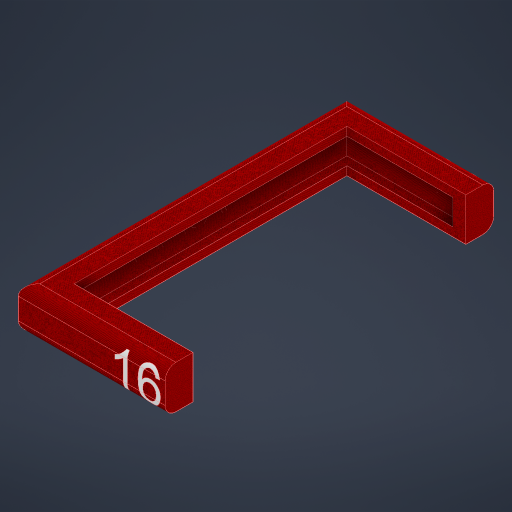
# Autodesk Inventor part: BUMP_005_BumperCloth
Saved by Autodesk Inventor 2024.2 (Build 282272000, 272)
## iProperties
Created: 2024-08-07
Part Number: BUMP_005_BumperCloth
Material: 1000 Denier Nylon Cordura
Document SubType Name: Modeling
Designer: Bryan
Density: 1 g/cm^3
Appearance: Default(1)
Mass: 229.5 g
Surface Area: 11381.8 cm^2
Volume: 229.5 cm^3
Author: Bryan
Autodesk Inventor part; units mm, degrees
ref_plane "YZ Plane" through (0, 0, 0) normal (1, 0, 0) x (0, 1, 0)
ref_plane "XZ Plane" through (0, 0, 0) normal (0, 1, 0) x (-1, 0, 0)
ref_plane "XY Plane" through (0, 0, 0) normal (0, 0, 1) x (1, 0, 0)
sketch "Sketch2" plane through (0, 0, 0) normal (1, 0, 0) x (0, 1, 0)
  line L0 (127, 0) -> (127, -82.55) construction
  line L1 (127, -82.55) -> (0, -82.55) construction
  line L2 (0, -82.55) -> (0, 0) construction
  circle A0 centre (95.25, -50.8) radius 31.75 construction
  circle A1 centre (31.75, -50.8) radius 31.75 construction
  arc A2 (95.25, -82.55) -> (127, -50.8) centre (95.25, -50.8) ccw
  arc A3 (0, -50.8) -> (31.75, -82.55) centre (31.75, -50.8) ccw
  line L3 (31.75, -82.55) -> (95.25, -82.55)
  line L4 (0, -50.8) -> (0, 0)
  line L5 (127, -50.8) -> (127, 0)
  line L6 (127, 0) -> (101.6, 0)
  line L7 (0, 0) -> (25.4, 0)
  line L8 (101.6, 0.4) -> (127.4, 0.4)
  line L9 (127.4, 0.4) -> (127.4, -50.8)
  arc A4 (95.25, -82.95) -> (127.4, -50.8) centre (95.25, -50.8) ccw
  line L10 (95.25, -82.95) -> (31.75, -82.95)
  arc A5 (-0.4, -50.8) -> (31.75, -82.95) centre (31.75, -50.8) ccw
  line L11 (-0.4, -50.8) -> (-0.4, 0.4)
  line L12 (-0.4, 0.4) -> (25.4, 0.4)
  line L13 (127, 0) -> (0, -82.55) construction
  line L14 (0, 0) -> (127, -82.55) construction
  line L15 (101.6, 0.4) -> (101.6, 0)
  line L16 (25.4, 0.4) -> (25.4, 0)
  point P0 (63.5, -41.275)
  dimension "d1" = 82.55
  dimension "d2" = 127
  dimension "d3" = 63.5
  dimension "d4" = 25.4
  dimension "d5" = 25.4
  dimension "d6" = 127
  dimension "d7" = 0.4
  constraints: 34 end point, 12 point on circle, 7 tangent, 6 centre point, 4 point on line, 4 vertical, 3 concentric, 3 horizontal, 1 equal radius, 1 midpoint, 1 parallel, 6 other
  measures "d1" distance of L0.start L0.end
  measures "d2" distance of L2.end L0.start
  measures "d3" diameter of A0
  measures "d4" distance of L0.start L6.end
  measures "d5" distance of L2.end L7.end
  measures "d6" distance of L0.end L1.end
  measures "d7" distance between parallel lines of L6 L8
sketch3d "3D Sketch1"
  line L0 (0, 63.5, -41.275) -> (-395.2875, 63.5, -41.275)
  line L1 (-395.2875, 63.5, -41.275) -> (-395.2875, 63.5, 854.075)
  line L2 (-395.2875, 63.5, 854.075) -> (0, 63.5, 854.075)
  dimension "d10" = 395.2875
  dimension "d11" = 895.35
sweep "Sweep1" add profiles "Sketch2" path "3D Sketch1"
sketch "Sketch3" plane through (0, 31.75, 895.35) normal (1, 0, 0) x (0, 0, -1)
  line L0 (895.35, -31.75) -> (895.35, -6.35) projected
  line L1 (895.35, -6.35) -> (894.95, -6.35) projected
  line L2 (894.95, -6.35) -> (894.95, -32.15) projected
  line L3 (894.95, -32.15) -> (946.15, -32.15) projected
  arc A0 (946.15, -32.15) -> (978.3, 0) centre (946.15, 0) ccw projected
  line L4 (978.3, 0) -> (978.3, 63.5) projected
  arc A1 (978.3, 63.5) -> (946.15, 95.65) centre (946.15, 63.5) ccw projected
  line L5 (946.15, 95.65) -> (894.95, 95.65) projected
  line L6 (894.95, 95.65) -> (894.95, 69.85) projected
  line L7 (894.95, 69.85) -> (895.35, 69.85) projected
  line L8 (895.35, 69.85) -> (895.35, 95.25) projected
  line L9 (895.35, 95.25) -> (946.15, 95.25) projected
  arc A2 (977.9, 63.5) -> (946.15, 95.25) centre (946.15, 63.5) ccw projected
  line L10 (977.9, 63.5) -> (977.9, 0) projected
  arc A3 (946.15, -31.75) -> (977.9, 0) centre (946.15, 0) ccw projected
  line L11 (946.15, -31.75) -> (895.35, -31.75) projected
  line L12 (894.95, 69.85) -> (894.95, -6.35)
  line L13 (82.55, -6.35) -> (82.55, -31.75) projected
  line L14 (82.55, -31.75) -> (31.75, -31.75) projected
  arc A4 (0, 0) -> (31.75, -31.75) centre (31.75, 0) ccw projected
  line L15 (0, 0) -> (0, 63.5) projected
  arc A5 (31.75, 95.25) -> (0, 63.5) centre (31.75, 63.5) ccw projected
  line L16 (31.75, 95.25) -> (82.55, 95.25) projected
  line L17 (82.55, 95.25) -> (82.55, 69.85) projected
  line L18 (82.55, 69.85) -> (82.95, 69.85) projected
  line L19 (82.95, 69.85) -> (82.95, 95.65) projected
  line L20 (82.95, 95.65) -> (31.75, 95.65) projected
  arc A6 (31.75, 95.65) -> (-0.4, 63.5) centre (31.75, 63.5) ccw projected
  line L21 (-0.4, 63.5) -> (-0.4, 0) projected
  arc A7 (-0.4, 0) -> (31.75, -32.15) centre (31.75, 0) ccw projected
  line L22 (31.75, -32.15) -> (82.95, -32.15) projected
  line L23 (82.95, -32.15) -> (82.95, -6.35) projected
  line L24 (82.95, -6.35) -> (82.55, -6.35) projected
  line L25 (82.95, 69.85) -> (82.95, -6.35)
  constraints: 4 end point, 2 vertical
extrude "Extrusion1" add sketch "Sketch3" along normal blind 0.4
sketch "Sketch4" plane through (-353.6125, 101.6, 812.4) normal (0, 0, -1) x (-1, 0, 0)
  line L0 (0, 0) -> (-353.6125, 0) projected
  line L1 (-353.6125, -76.2) -> (-353.6125, 0) projected
  line L2 (0, -76.2) -> (-353.6125, -76.2) projected
  line L3 (-315.5125, 0) -> (-315.5125, -76.2)
  point P0 (-353.6125, -101.6)
  dimension "d16" = 38.1
  constraints: 2 end point, 2 point on line, 1 vertical
  measures "d16" distance between parallel lines of L1 L3
extrude "Extrusion2" add sketch "Sketch4" against normal blind 0.4
sketch "Sketch6" plane through (0, 31.75, 895.35) normal (1, 0, 0) x (0, 0, -1)
  line L0 (82.95, 95.65) -> (31.75, 95.65) projected
  arc A0 (31.75, 95.65) -> (-0.4, 63.5) centre (31.75, 63.5) ccw construction
  line L1 (-0.4, 63.5) -> (-0.4, 0) projected
  arc A1 (-0.4, 0) -> (31.75, -32.15) centre (31.75, 0) ccw projected
  line L2 (31.75, -32.15) -> (82.95, -32.15) projected
  line L3 (82.95, -32.15) -> (82.95, 95.65) projected
  arc A2 (31.75, 95.75) -> (-0.5, 63.5) centre (31.75, 63.5) ccw
  line L4 (31.75, 95.75) -> (83.05, 95.75)
  line L5 (83.05, 95.75) -> (83.05, -32.25)
  line L6 (83.05, -32.25) -> (31.75, -32.25)
  arc A3 (-0.5, 0) -> (31.75, -32.25) centre (31.75, 0) ccw
  line L7 (-0.5, 0) -> (-0.5, 63.5)
  arc A4 (31.75, 146.55) -> (-51.3, 63.5) centre (31.75, 63.5) ccw
  line L8 (31.75, 146.55) -> (133.85, 146.55)
  line L9 (133.85, 146.55) -> (133.85, -83.05)
  line L10 (133.85, -83.05) -> (31.75, -83.05)
  arc A5 (-51.3, 0) -> (31.75, -83.05) centre (31.75, 0) ccw
  line L11 (-51.3, 0) -> (-51.3, 63.5)
  point P0 (895.35, -31.75)
  dimension "d22" = 0.1
  dimension "d51" = 50.8
  constraints: 16 end point, 8 point on circle, 4 centre point, 10 other
  measures "d22" radial gap between concentric circles of A0 A2
  measures "d51" radial gap between concentric circles of A2 A4
ref_plane "Work Plane1" through (-436.9625, 31.75, 895.85) normal (0, 0, 1) x (1, 0, 0)
sketch "Sketch5" plane through (-353.6125, -0.4, 0.4) normal (0, 0, 1) x (1, 0, 0)
  line L0 (353.6125, 102) -> (0, 102) projected
  line L1 (353.6125, 102) -> (353.6125, 25.8) projected
  line L2 (353.6125, 25.8) -> (0, 25.8) projected
  line L3 (315.5125, 102) -> (315.5125, 25.8)
  point P0 (353.6125, 0.4)
  dimension "d19" = 38.1
  constraints: 2 end point, 2 point on line, 1 vertical
  measures "d19" distance between parallel lines of L1 L3
extrude "Extrusion3" add sketch "Sketch5" against normal blind 0.4
sketch "Sketch9" plane through (-436.9625, 31.75, 895.85) normal (0, 0, 1) x (1, 0, 0)
  line L0 (272.2625, 82.95) -> (424.6625, 82.95) construction
  line L1 (424.6625, 82.95) -> (424.6625, -18.65) construction
  line L2 (424.6625, -18.65) -> (272.2625, -18.65) construction
  line L3 (272.2625, -18.65) -> (272.2625, 82.95) construction
  line L4 (32.15, 95.65) -> (437.3625, 95.65) projected
  line L5 (437.3625, 63.5) -> (437.3625, 0) projected
  line L6 (325.0759, -19.0372) -> (312.6082, -19.0372)
  line L7 (312.6082, -19.0372) -> (312.6082, 60.4152)
  spline S0 degree 2 poles (312.6082, 60.4152) (308.1168, 56.1561) (293.4808, 47.5604) (287.6729, 45.3921) knots 0 0 0 1 2 2 2
  line L8 (287.6729, 45.3921) -> (287.6729, 57.4726)
  spline S1 degree 2 poles (287.6729, 57.4726) (298.1271, 62.3512) (313.7698, 76.3677) (317.0223, 82.95) knots 0 0 0 1 2 2 2
  line L9 (317.0223, 82.95) -> (325.0759, 82.95)
  line L10 (325.0759, 82.95) -> (325.0759, -19.0372)
  line L11 (421.8747, 57.6274) -> (409.4844, 56.6207)
  spline S2 degree 2 poles (409.4844, 56.6207) (407.7808, 63.9774) (404.7607, 67.3848) knots 0 0 0 1 1 1
  spline S3 degree 2 poles (404.7607, 67.3848) (399.6497, 72.728) (392.2155, 72.728) knots 0 0 0 1 1 1
  spline S4 degree 2 poles (392.2155, 72.728) (386.2527, 72.728) (381.7613, 69.3982) knots 0 0 0 1 1 1
  spline S5 degree 2 poles (381.7613, 69.3982) (375.8759, 65.139) (369.0613, 48.5671) (368.9064, 33.3116) knots 0 0 0 1 2 2 2
  spline S6 degree 2 poles (368.9064, 33.3116) (373.3979, 40.2037) (386.4851, 46.8634) (393.6094, 46.8634) knots 0 0 0 1 2 2 2
  spline S7 degree 2 poles (393.6094, 46.8634) (406.0771, 46.8634) (423.6558, 28.5104) (423.6558, 13.9518) knots 0 0 0 1 2 2 2
  spline S8 degree 2 poles (423.6558, 13.9518) (423.6558, 4.4268) (415.3698, -11.9902) (400.9662, -20.7409) (391.8284, -20.7409) knots 0 0 0 1 2 3 3 3
  spline S9 degree 2 poles (391.8284, -20.7409) (376.1857, -20.7409) (356.5162, 2.1811) (356.5162, 28.5104) knots 0 0 0 1 2 2 2
  spline S10 degree 2 poles (356.5162, 28.5104) (356.5162, 57.9372) (367.4351, 71.3341) knots 0 0 0 1 1 1
  spline S11 degree 2 poles (367.4351, 71.3341) (376.8826, 82.95) (392.9899, 82.95) knots 0 0 0 1 1 1
  spline S12 degree 2 poles (392.9899, 82.95) (404.993, 82.95) (420.3259, 69.4756) (421.8747, 57.6274) knots 0 0 0 1 2 2 2
  spline S13 degree 2 poles (370.8424, 13.8744) (370.8424, 7.4469) (376.3405, -4.3238) (386.0979, -10.5189) (391.5186, -10.5189) knots 0 0 0 1 2 3 3 3
  spline S14 degree 2 poles (391.5186, -10.5189) (399.4948, -10.5189) (410.8009, 2.2585) (410.8009, 13.1774) knots 0 0 0 1 2 2 2
  spline S15 degree 2 poles (410.8009, 13.1774) (410.8009, 23.7091) (399.6497, 35.8671) (391.054, 35.8671) knots 0 0 0 1 2 2 2
  spline S16 degree 2 poles (391.054, 35.8671) (382.6131, 35.8671) (370.8424, 23.7091) (370.8424, 13.8744) knots 0 0 0 1 2 2 2
  point P0 (436.9625, -31.75)
  dimension "d31" = 101.6
  dimension "d32" = 152.4
  dimension "d33" = 12.7
  dimension "d34" = 12.7
  constraints: 2 other
  measures "d31" distance of L0.end L1.end
  measures "d32" distance of L0.start L0.end
  measures "d33" distance between parallel lines of L4 L0
  measures "d34" distance between parallel lines of L5 L1
extrude "Extrusion4" add sketch "Sketch9" against normal blind 12.7
ref_plane "Work Plane2" through (-437.0625, 31.75, -82.95) normal (-1, 0, 0) x (0, 0, 1)
sketch "Sketch10" plane through (-437.0625, 31.75, -82.95) normal (-1, 0, 0) x (0, 0, 1)
  line L0 (324.25, 82.15) -> (654.45, 82.15) construction
  line L1 (654.45, 82.15) -> (654.45, -19.45) construction
  line L2 (654.45, -19.45) -> (324.25, -19.45) construction
  line L3 (324.25, -19.45) -> (324.25, 82.15) construction
  line L4 (32.15, -32.15) -> (946.55, -32.15) projected
  line L5 (0, 63.5) -> (0, 0) projected
  line L6 (978.7, 63.5) -> (978.7, 0) projected
  line L7 (377.0634, -19.8372) -> (364.5957, -19.8372)
  line L8 (364.5957, -19.8372) -> (364.5957, 59.6152)
  spline S0 degree 2 poles (364.5957, 59.6152) (360.1043, 55.3561) (345.4683, 46.7604) (339.6604, 44.5921) knots 0 0 0 1 2 2 2
  line L9 (339.6604, 44.5921) -> (339.6604, 56.6726)
  spline S1 degree 2 poles (339.6604, 56.6726) (350.1146, 61.5512) (365.7573, 75.5677) (369.0098, 82.15) knots 0 0 0 1 2 2 2
  line L10 (369.0098, 82.15) -> (377.0634, 82.15)
  line L11 (377.0634, 82.15) -> (377.0634, -19.8372)
  line L12 (473.8622, 56.8274) -> (461.4719, 55.8207)
  spline S2 degree 2 poles (461.4719, 55.8207) (459.7683, 63.1774) (456.7482, 66.5848) knots 0 0 0 1 1 1
  spline S3 degree 2 poles (456.7482, 66.5848) (451.6372, 71.928) (444.203, 71.928) knots 0 0 0 1 1 1
  spline S4 degree 2 poles (444.203, 71.928) (438.2402, 71.928) (433.7488, 68.5982) knots 0 0 0 1 1 1
  spline S5 degree 2 poles (433.7488, 68.5982) (427.8634, 64.339) (421.0488, 47.7671) (420.8939, 32.5116) knots 0 0 0 1 2 2 2
  spline S6 degree 2 poles (420.8939, 32.5116) (425.3854, 39.4037) (438.4726, 46.0634) (445.5969, 46.0634) knots 0 0 0 1 2 2 2
  spline S7 degree 2 poles (445.5969, 46.0634) (458.0646, 46.0634) (475.6433, 27.7104) (475.6433, 13.1518) knots 0 0 0 1 2 2 2
  spline S8 degree 2 poles (475.6433, 13.1518) (475.6433, 3.6268) (467.3573, -12.7902) (452.9537, -21.5409) (443.8159, -21.5409) knots 0 0 0 1 2 3 3 3
  spline S9 degree 2 poles (443.8159, -21.5409) (428.1732, -21.5409) (408.5037, 1.3811) (408.5037, 27.7104) knots 0 0 0 1 2 2 2
  spline S10 degree 2 poles (408.5037, 27.7104) (408.5037, 57.1372) (419.4226, 70.5341) knots 0 0 0 1 1 1
  spline S11 degree 2 poles (419.4226, 70.5341) (428.8701, 82.15) (444.9774, 82.15) knots 0 0 0 1 1 1
  spline S12 degree 2 poles (444.9774, 82.15) (456.9805, 82.15) (472.3134, 68.6756) (473.8622, 56.8274) knots 0 0 0 1 2 2 2
  spline S13 degree 2 poles (422.8299, 13.0744) (422.8299, 6.6469) (428.328, -5.1238) (438.0854, -11.3189) (443.5061, -11.3189) knots 0 0 0 1 2 3 3 3
  spline S14 degree 2 poles (443.5061, -11.3189) (451.4823, -11.3189) (462.7884, 1.4585) (462.7884, 12.3774) knots 0 0 0 1 2 2 2
  spline S15 degree 2 poles (462.7884, 12.3774) (462.7884, 22.9091) (451.6372, 35.0671) (443.0415, 35.0671) knots 0 0 0 1 2 2 2
  spline S16 degree 2 poles (443.0415, 35.0671) (434.6006, 35.0671) (422.8299, 22.9091) (422.8299, 13.0744) knots 0 0 0 1 2 2 2
  line L13 (553.4695, -7.8342) -> (553.4695, -19.8372)
  line L14 (553.4695, -19.8372) -> (486.3299, -19.8372)
  spline S17 degree 2 poles (486.3299, -19.8372) (486.175, -15.3457) (487.8012, -11.164) knots 0 0 0 1 1 1
  spline S18 degree 2 poles (487.8012, -11.164) (490.3567, -4.272) (501.6628, 8.9701) (512.3494, 17.7207) knots 0 0 0 1 2 2 2
  spline S19 degree 2 poles (512.3494, 17.7207) (528.8439, 31.35) (540.4598, 47.1476) (540.4598, 54.2719) knots 0 0 0 1 2 2 2
  spline S20 degree 2 poles (540.4598, 54.2719) (540.4598, 61.7061) (529.8506, 71.8506) (521.3323, 71.8506) knots 0 0 0 1 2 2 2
  spline S21 degree 2 poles (521.3323, 71.8506) (512.3494, 71.8506) (501.5854, 61.0091) (501.5079, 51.4841) knots 0 0 0 1 2 2 2
  line L15 (501.5079, 51.4841) -> (488.653, 52.8006)
  spline S22 degree 2 poles (488.653, 52.8006) (489.9695, 67.1268) (507.161, 82.15) (521.6421, 82.15) knots 0 0 0 1 2 2 2
  spline S23 degree 2 poles (521.6421, 82.15) (536.278, 82.15) (553.3146, 65.9652) (553.3146, 53.9622) knots 0 0 0 1 2 2 2
  spline S24 degree 2 poles (553.3146, 53.9622) (553.3146, 47.8445) (548.3585, 36.0738) (536.7427, 23.064) (523.3457, 11.6805) knots 0 0 0 1 2 3 3 3
  spline S25 degree 2 poles (523.3457, 11.6805) (512.1171, 2.3104) (505.7671, -4.4268) (503.6762, -7.8342) knots 0 0 0 1 2 2 2
  line L16 (503.6762, -7.8342) -> (553.4695, -7.8342)
  line L17 (632.3799, -7.8342) -> (632.3799, -19.8372)
  line L18 (632.3799, -19.8372) -> (565.2402, -19.8372)
  spline S26 degree 2 poles (565.2402, -19.8372) (565.0854, -15.3457) (566.7116, -11.164) knots 0 0 0 1 1 1
  spline S27 degree 2 poles (566.7116, -11.164) (569.2671, -4.272) (580.5732, 8.9701) (591.2598, 17.7207) knots 0 0 0 1 2 2 2
  spline S28 degree 2 poles (591.2598, 17.7207) (607.7543, 31.35) (619.3701, 47.1476) (619.3701, 54.2719) knots 0 0 0 1 2 2 2
  spline S29 degree 2 poles (619.3701, 54.2719) (619.3701, 61.7061) (608.761, 71.8506) (600.2427, 71.8506) knots 0 0 0 1 2 2 2
  spline S30 degree 2 poles (600.2427, 71.8506) (591.2598, 71.8506) (580.4957, 61.0091) (580.4183, 51.4841) knots 0 0 0 1 2 2 2
  line L19 (580.4183, 51.4841) -> (567.5634, 52.8006)
  spline S31 degree 2 poles (567.5634, 52.8006) (568.8799, 67.1268) (586.0713, 82.15) (600.5524, 82.15) knots 0 0 0 1 2 2 2
  spline S32 degree 2 poles (600.5524, 82.15) (615.1884, 82.15) (632.225, 65.9652) (632.225, 53.9622) knots 0 0 0 1 2 2 2
  spline S33 degree 2 poles (632.225, 53.9622) (632.225, 47.8445) (627.2689, 36.0738) (615.653, 23.064) (602.2561, 11.6805) knots 0 0 0 1 2 3 3 3
  spline S34 degree 2 poles (602.2561, 11.6805) (591.0274, 2.3104) (584.6774, -4.4268) (582.5866, -7.8342) knots 0 0 0 1 2 2 2
  line L20 (582.5866, -7.8342) -> (632.3799, -7.8342)
  point P0 (82.95, -31.75)
  point P1 (489.35, 82.15)
  dimension "d38" = 330.2
  dimension "d39" = 101.6
  dimension "d40" = 12.7
  dimension "d41" = 489.35
  dimension "d56" = 978.7
  constraints: 1 midpoint, 2 other
  measures "d38" distance of L0.start L0.end
  measures "d39" distance of L2.end L0.start
  measures "d40" distance between parallel lines of L4 L2
  measures "d41" distance from line of L5 point (489.35, 82.15)
  measures "d56" distance between parallel lines of L6 L5
extrude "Extrusion5" add sketch "Sketch10" against normal blind 12.7
ref_plane "Work Plane3" through (-436.9625, 31.75, -83.05) normal (0, 0, -1) x (-1, 0, 0)
sketch "Sketch11" plane through (-436.9625, 31.75, -83.05) normal (0, 0, -1) x (-1, 0, 0)
  line L0 (-424.6625, 82.55) -> (-272.2625, 82.55) construction
  line L1 (-272.2625, 82.55) -> (-272.2625, -19.05) construction
  line L2 (-272.2625, -19.05) -> (-424.6625, -19.05) construction
  line L3 (-424.6625, -19.05) -> (-424.6625, 82.55) construction
  line L4 (-436.9625, 95.25) -> (-32.15, 95.25) projected
  line L5 (-437.3625, 0) -> (-437.3625, 63.5) projected
  line L6 (-353.2637, -7.4342) -> (-353.2637, -19.4372)
  line L7 (-353.2637, -19.4372) -> (-420.4034, -19.4372)
  spline S0 degree 2 poles (-420.4034, -19.4372) (-420.5582, -14.9457) (-418.932, -10.764) knots 0 0 0 1 1 1
  spline S1 degree 2 poles (-418.932, -10.764) (-416.3765, -3.872) (-405.0704, 9.3701) (-394.3838, 18.1207) knots 0 0 0 1 2 2 2
  spline S2 degree 2 poles (-394.3838, 18.1207) (-377.8893, 31.75) (-366.2735, 47.5476) (-366.2735, 54.6719) knots 0 0 0 1 2 2 2
  spline S3 degree 2 poles (-366.2735, 54.6719) (-366.2735, 62.1061) (-376.8826, 72.2506) (-385.4009, 72.2506) knots 0 0 0 1 2 2 2
  spline S4 degree 2 poles (-385.4009, 72.2506) (-394.3838, 72.2506) (-405.1479, 61.4091) (-405.2253, 51.8841) knots 0 0 0 1 2 2 2
  line L8 (-405.2253, 51.8841) -> (-418.0802, 53.2006)
  spline S5 degree 2 poles (-418.0802, 53.2006) (-416.7637, 67.5268) (-399.5723, 82.55) (-385.0912, 82.55) knots 0 0 0 1 2 2 2
  spline S6 degree 2 poles (-385.0912, 82.55) (-370.4552, 82.55) (-353.4186, 66.3652) (-353.4186, 54.3622) knots 0 0 0 1 2 2 2
  spline S7 degree 2 poles (-353.4186, 54.3622) (-353.4186, 48.2445) (-358.3747, 36.4738) (-369.9905, 23.464) (-383.3875, 12.0805) knots 0 0 0 1 2 3 3 3
  spline S8 degree 2 poles (-383.3875, 12.0805) (-394.6162, 2.7104) (-400.9662, -4.0268) (-403.057, -7.4342) knots 0 0 0 1 2 2 2
  line L9 (-403.057, -7.4342) -> (-353.2637, -7.4342)
  line L10 (-274.3534, -7.4342) -> (-274.3534, -19.4372)
  line L11 (-274.3534, -19.4372) -> (-341.493, -19.4372)
  spline S9 degree 2 poles (-341.493, -19.4372) (-341.6479, -14.9457) (-340.0216, -10.764) knots 0 0 0 1 1 1
  spline S10 degree 2 poles (-340.0216, -10.764) (-337.4662, -3.872) (-326.1601, 9.3701) (-315.4735, 18.1207) knots 0 0 0 1 2 2 2
  spline S11 degree 2 poles (-315.4735, 18.1207) (-298.979, 31.75) (-287.3631, 47.5476) (-287.3631, 54.6719) knots 0 0 0 1 2 2 2
  spline S12 degree 2 poles (-287.3631, 54.6719) (-287.3631, 62.1061) (-297.9723, 72.2506) (-306.4906, 72.2506) knots 0 0 0 1 2 2 2
  spline S13 degree 2 poles (-306.4906, 72.2506) (-315.4735, 72.2506) (-326.2375, 61.4091) (-326.3149, 51.8841) knots 0 0 0 1 2 2 2
  line L12 (-326.3149, 51.8841) -> (-339.1698, 53.2006)
  spline S14 degree 2 poles (-339.1698, 53.2006) (-337.8534, 67.5268) (-320.6619, 82.55) (-306.1808, 82.55) knots 0 0 0 1 2 2 2
  spline S15 degree 2 poles (-306.1808, 82.55) (-291.5448, 82.55) (-274.5082, 66.3652) (-274.5082, 54.3622) knots 0 0 0 1 2 2 2
  spline S16 degree 2 poles (-274.5082, 54.3622) (-274.5082, 48.2445) (-279.4643, 36.4738) (-291.0802, 23.464) (-304.4771, 12.0805) knots 0 0 0 1 2 3 3 3
  spline S17 degree 2 poles (-304.4771, 12.0805) (-315.7058, 2.7104) (-322.0558, -4.0268) (-324.1466, -7.4342) knots 0 0 0 1 2 2 2
  line L13 (-324.1466, -7.4342) -> (-274.3534, -7.4342)
  point P0 (-436.9625, -31.75)
  dimension "d45" = 152.4
  dimension "d46" = 101.6
  dimension "d47" = 12.7
  dimension "d48" = 12.7
  constraints: 2 other
  measures "d45" distance of L0.start L0.end
  measures "d46" distance of L0.end L1.end
  measures "d47" distance between parallel lines of L4 L0
  measures "d48" distance between parallel lines of L3 L5
extrude "Extrusion6" add sketch "Sketch11" against normal blind 12.7
sketch3d "3D Sketch1 for Sweep2"
  line L0 (0, 63.5, 854.075) -> (-395.2875, 63.5, 854.075)
  line L1 (-395.2875, 63.5, 854.075) -> (-395.2875, 63.5, -41.275)
  line L2 (-395.2875, 63.5, -41.275) -> (0, 63.5, -41.275)
  dimension "d10" = 395.2875
  dimension "d11" = 895.35
sweep "Sweep2" cut profiles "Sketch6" path "3D Sketch1 for Sweep2"
sketch "Sketch12" plane through (0, 31.75, 895.35) normal (-1, 0, 0) x (0, 0, 1)
  line L0 (-895.35, -31.75) -> (-895.35, 95.25) projected
  line L1 (-895.35, 95.25) -> (-946.15, 95.25) projected
  arc A0 (-946.15, 95.25) -> (-977.9, 63.5) centre (-946.15, 63.5) ccw projected
  line L2 (-977.9, 63.5) -> (-977.9, 0) projected
  arc A1 (-977.9, 0) -> (-946.15, -31.75) centre (-946.15, 0) ccw projected
  line L3 (-946.15, -31.75) -> (-895.35, -31.75) projected
sketch3d "3D Sketch1 for Sweep3"
  line L0 (0, 63.5, -41.275) -> (-395.2875, 63.5, -41.275)
  line L1 (-395.2875, 63.5, -41.275) -> (-395.2875, 63.5, 854.075)
  line L2 (-395.2875, 63.5, 854.075) -> (0, 63.5, 854.075)
  dimension "d10" = 395.2875
  dimension "d11" = 895.35
sweep "Sweep3" cut profiles "Sketch12" path "3D Sketch1 for Sweep3"
equation "\"d41\" = 0.5 * d56"
body "Solid1"
